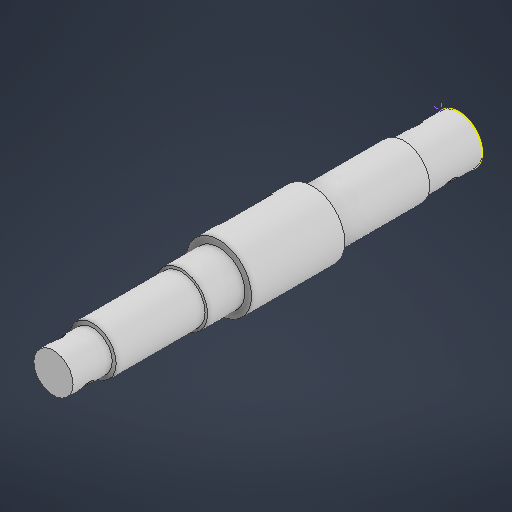
# Autodesk Inventor part: laborator2 final
Saved by Autodesk Inventor 2026.2 (Build 302298010, 298A)
## iProperties
Created: 2026-03-03
Part Number: laborator2 final
Material: Generic
Document SubType Name: Modeling
Designer: Ramen
Density: 1 g/cm^3
Appearance: Default
Author: Ramen
Autodesk Inventor part; units mm, degrees
ref_plane "YZ Plane" through (0, 0, 0) normal (1, 0, 0) x (0, 1, 0)
ref_plane "XZ Plane" through (0, 0, 0) normal (0, 1, 0) x (-1, 0, 0)
sketch "Sketch1" plane through (0, 0, 0) normal (0, 1, 0) x (-1, 0, 0)
  line L0 (0, 0) -> (0, -155)
  line L1 (0, -155) -> (9, -155)
  line L2 (9, -155) -> (9, -134)
  line L3 (9, -134) -> (10, -134)
  line L4 (10, -134) -> (10, -99)
  line L5 (10, -99) -> (12.5, -99)
  line L6 (12.5, -99) -> (12.5, -63.3)
  line L7 (12.5, -63.3) -> (10, -63.3)
  line L8 (10, -63.3) -> (10, -49)
  line L9 (10, -49) -> (9, -49)
  line L10 (9, -49) -> (9, -15)
  line L11 (9, -15) -> (7.5, -15)
  line L12 (7.5, -15) -> (7.5, 0)
  line L13 (7.5, 0) -> (0, 0)
  dimension "d1" = 155
  dimension "d2" = 9
  dimension "d3" = 21
  dimension "d4" = 1
  dimension "d5" = 35
  dimension "d6" = 2.5
  dimension "d7" = 35.7
  dimension "d8" = 2.5
  dimension "d9" = 14.3
  dimension "d10" = 1
  dimension "d11" = 34
  dimension "d12" = 1.5
  dimension "d13" = 15
  constraints: 28 end point, 7 perpendicular, 2 horizontal, 2 point on line, 2 vertical
  measures "d1" distance of L0.start L0.end
  measures "d2" distance of L0.end L1.end
  measures "d3" distance of L1.end L2.end
  measures "d4" distance of L2.end L3.end
  measures "d5" distance of L3.end L4.end
  measures "d6" distance of L4.end L5.end
  measures "d7" distance of L5.end L6.end
  measures "d8" distance of L6.end L7.end
  measures "d9" distance of L7.end L8.end
  measures "d10" distance of L8.end L9.end
  measures "d11" distance of L9.end L10.end
  measures "d12" distance of L10.end L11.end
  measures "d13" distance of L11.end L12.end
revolve "Revolution1" add sketch "Sketch1" angle 360 about axis through (0, 0, 0) along (0, 0, -1)
sketch "Sketch2" plane through (0, 0, -155) normal (0, 0, -1) x (-1, 0, 0)
  circle A0 centre (0, 0) radius 9 projected
  circle A1 centre (0, 0) radius 7.5 projected
  point P0 (6.6798, 6.0316)
  constraints: 1 coincident, 2 other
ref_plane "Work Plane1" through (-6.6798, 6.0316, -155) normal (-0.7421989, 0.6701796, 0) x (-0.6701796, -0.7421989, 0)
sketch "Sketch3" plane through (-6.6798, 6.0316, -155) normal (-0.7421989, 0.6701796, 0) x (-0.6701796, -0.7421989, 0)
  line L0 (-9, 0) -> (9, 0) projected
  circle A0 centre (0, 10) radius 2.5
  point P0 (0, 155)
  dimension "d17" = 5
  dimension "d18" = 10
  constraints: 1 centre point
  measures "d17" diameter of A0
  measures "d18" distance from line of L0 A0.centre
extrude "Extrusion1" cut sketch "Sketch3" against normal through all
ref_plane "Work Plane2" through (0, 0, 0) normal (-0.6701796, -0.7421989, 0) x (0, 0, 1)
sketch "Sketch4" plane through (0, 0, 0) normal (-0.6701796, -0.7421989, 0) x (0, 0, 1)
  line L0 (-99, 12.5) -> (-99, -12.5) projected
  line L1 (-57, 0) -> (-57, 17.3) construction
  line L2 (-81, 17.2999) -> (-81, -8.0858) construction
  line L3 (-57, 17.3) -> (-99, 17.3) construction
  arc A0 (-90.8975, 12.5) -> (-71.1025, 12.5) centre (-81, 17.2999) ccw
  line L4 (-63.3, 12.5) -> (-99, 12.5) projected
  point P0 (0, 0)
  dimension "d22" = 17.3
  dimension "d24" = 18
  dimension "d25" = 24
  dimension "d27" = 11
  dimension "d28" = 19.795
  constraints: 6 end point, 3 point on line, 2 coincident, 2 point on circle, 2 vertical, 1 centre point, 1 horizontal
  measures "d22" distance of L1.start L1.end
  measures "d24" distance from line of L0.start L2
  measures "d25" distance from line of L2 L1.start
  measures "d27" radius of A0
  measures "d28" distance of A0.start A0.end
extrude "Extrusion2" cut sketch "Sketch4" along normal mid plane 6
sketch "Sketch5" plane through (0, 0, 0) normal (-0.6701796, -0.7421989, 0) x (0, 0, 1)
  line L0 (-15, 9) -> (-15, -9) projected
  line L1 (-15, 9) -> (-7, 9) construction
  line L2 (-15, 9) -> (-49, 9) construction
  line L3 (-7, 9) -> (-7, 7.5) construction
  line L4 (0, 7.5) -> (-15, 7.5) construction
  line L5 (-7, 7.5) -> (-9.65, 7.5) construction
  line L6 (-7, 7.5) -> (-7, -7.5) construction
  line L7 (0, -7.5) -> (-15, -7.5) construction
  line L8 (-7, -7.5) -> (-9.5, -7.5) construction
  line L9 (-9.5, -7.5) -> (-9.65, 7.5) construction
  line L10 (-7, 7.5) -> (-9.65, 7.5)
  line L11 (-9.5, -7.5) -> (-7, -7.5)
  line L12 (-7, 7.5) -> (-7, -7.5)
  line L13 (-9.5, -7.5) -> (-9.65, 7.5)
  point P0 (0, 0)
  dimension "d31" = 8
  dimension "d41" = 2.65
  dimension "d42" = 2.5
  constraints: 20 end point, 5 collinear, 4 point on line, 2 vertical
  measures "d31" distance of L0.start L1.end
  measures "d41" distance of L3.end L5.end
  measures "d42" distance of L6.end L8.end
revolve "Revolution2" cut sketch "Sketch5" angle 360 about axis through (-5.5665, 5.0263, -7) along (0.7421989, -0.6701796, 0)
body "Solid1"
